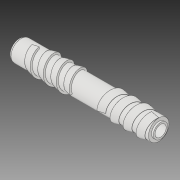
# Autodesk Inventor part: Dribblerschnecke
Saved by Autodesk Inventor 2019.4 (Build 234330000, 330)
## iProperties
Part Number: Dribblerschnecke
Material: Acetalharz, weiß
Document SubType Name: Modeling
Designer: rYan
Mass: 7.87255 g
Surface Area: 45.3022 cm^2
Volume: 5.5246 cm^3
Density: 1.425 g/cm^3
Appearance: Glatt - weiß
Author: rYan
Autodesk Inventor part; units mm, degrees
ref_plane "YZ Plane" through (0, 0, 0) normal (1, 0, 0) x (0, 1, 0)
ref_plane "XZ Plane" through (0, 0, 0) normal (0, 1, 0) x (-1, 0, 0)
ref_plane "XY Plane" through (0, 0, 0) normal (0, 0, 1) x (1, 0, 0)
sketch "Skizze1" plane through (0, 0, 0) normal (1, 0, 0) x (0, 1, 0)
  circle A0 centre (0, 0) radius 3
  circle A1 centre (0, 0) radius 5.5
  dimension "d0" = 6
  dimension "d1" = 11
  constraints: 2 centre point, 2 coincident
  measures "d0" diameter of A0
  measures "d1" diameter of A1
extrude "Extrusion1" add sketch "Skizze1" along normal blind 34
sketch "Skizze3" plane through (0, 0, 0) normal (0, 1, 0) x (-1, 0, 0)
  line L0 (-34, 5.5) -> (-30, 5.5)
  line L1 (-30, 5.5) -> (-30.1763, 6.5)
  line L2 (-30.1763, 6.5) -> (-34, 5.6)
  line L3 (-34, 5.6) -> (-34, 5.5)
  line L4 (-34, 5.5) -> (-34, -5.5) construction
  line L5 (0, -5.5) -> (0, 5.5) construction
  point P0 (0, 0)
  dimension "d16" = 4
  dimension "d17" = 80
  dimension "d18" = 1
  dimension "d19" = 0.1
  constraints: 8 end point, 1 horizontal, 1 vertical
  measures "d16" distance of L0.start L0.end
  measures "d17" angle of L1 L0
  measures "d18" distance from line of L0 L1.end
  measures "d19" distance of L2.end L0.start
coil "Spirale1" sketch "Skizze3" operation add axis through (-10, 0, 0) along (-1, 0, 0) pitch 7 turns 3.285714 hand left
mirror "Spiegeln1" about plane through (0, 0, 0) normal (1, 0, 0) of "Extrusion1", "Spirale1"
sketch "Skizze4" plane through (34, 0, 0) normal (1, 0, 0) x (0, 0, -1)
  circle A0 centre (0, 0) radius 3 projected
  circle A1 centre (0, 0) radius 3.9
  dimension "d23" = 7.8
  constraints: 1 centre point, 1 coincident
  measures "d23" diameter of A1
extrude "Extrusion2" add sketch "Skizze4" along normal blind 1
sketch "Skizze5" plane through (-34, 0, 0) normal (-1, 0, 0) x (0, 0, 1)
  circle A0 centre (0, 0) radius 3 projected
  circle A1 centre (0, 0) radius 3 projected
  circle A2 centre (0, 0) radius 5.5 projected
  point P0 (5.5, 0)
  constraints: 1 horizontal alignment
extrude "Extrusion3" add sketch "Skizze5" along normal blind 5.8
sketch "Skizze6" plane through (-39.8, 0, 0) normal (-1, 0, 0) x (0, 0, 1)
  circle A0 centre (0, 0) radius 3 projected
  circle A1 centre (0, 0) radius 5
  circle A2 centre (0, 0) radius 3.9 projected
  dimension "d31" = 10
  constraints: 1 centre point, 1 coincident, 1 concentric
  measures "d31" diameter of A1
extrude "Extrusion4" add sketch "Skizze6" along normal blind 1 contours A1 | A2
